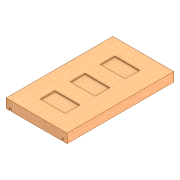
# Autodesk Inventor part: topplatform
Saved by Autodesk Inventor 2020 (Build 240168000, 168)
## iProperties
Created: 2021-06-22
Part Number: topplatform
Material: Generic
Document SubType Name: Modeling
Designer: Aidan Lee
Density: 1 g/cm^3
Appearance: Cherry - Natural Low Gloss
Author: Aidan Lee
Autodesk Inventor part; units mm, degrees
ref_plane "YZ Plane" through (0, 0, 0) normal (1, 0, 0) x (0, 1, 0)
ref_plane "XZ Plane" through (0, 0, 0) normal (0, 1, 0) x (-1, 0, 0)
ref_plane "XY Plane" through (0, 0, 0) normal (0, 0, 1) x (1, 0, 0)
sketch "Sketch1" plane through (0, 0, 0) normal (0, 0, 1) x (1, 0, 0)
  line L0 (0, 0) -> (120, 0)
  line L1 (120, 0) -> (120, 18)
  line L2 (120, 18) -> (0, 18)
  line L3 (0, 18) -> (0, 0)
  dimension "d0" = 18
  dimension "d1" = 120
  constraints: 8 end point, 2 parallel, 1 horizontal, 1 perpendicular
  measures "d0" distance of L2.end L0.start
  measures "d1" distance of L0.start L0.end
extrude "Extrusion1" add sketch "Sketch1" along normal blind 210
sketch "Sketch2" plane through (0, 0, 210) normal (0, 0, 1) x (1, 0, 0)
  line L0 (0, 0) -> (120, 0) projected
  line L1 (7, 0) -> (10, 0)
  line L2 (10, 0) -> (10, 5)
  line L3 (10, 5) -> (7, 5)
  line L4 (7, 5) -> (7, 0)
  line L5 (60, 0) -> (60, -17.5294) construction
  line L6 (113, 0) -> (110, 0)
  line L7 (110, 0) -> (110, 5)
  line L8 (110, 5) -> (113, 5)
  line L9 (113, 5) -> (113, 0)
  point P0 (110, 0)
  point P1 (113, 0)
  dimension "d4" = 3
  dimension "d5" = 5
  dimension "d26" = 100
  constraints: 18 end point, 4 symmetric about line, 2 parallel, 1 horizontal, 1 midpoint, 1 perpendicular, 1 point on line, 1 vertical
  measures "d4" distance of L2.end L3.end
  measures "d5" distance of L3.end L1.start
  measures "d26" distance between parallel lines of L7 L2
extrude "Extrusion2" cut sketch "Sketch2" against normal through all
sketch "Sketch3" plane through (0, 18, 0) normal (0, 1, 0) x (1, 0, 0)
  line L0 (35.5, -31.5) -> (84.5, -31.5)
  line L1 (84.5, -31.5) -> (84.5, -60.5)
  line L2 (84.5, -60.5) -> (35.5, -60.5)
  line L3 (35.5, -60.5) -> (35.5, -31.5)
  line L4 (35.5, -90.5) -> (84.5, -90.5)
  line L5 (84.5, -90.5) -> (84.5, -119.5)
  line L6 (84.5, -119.5) -> (35.5, -119.5)
  line L7 (35.5, -119.5) -> (35.5, -90.5)
  line L8 (35.5, -149.5) -> (84.5, -149.5)
  line L9 (84.5, -149.5) -> (84.5, -178.5)
  line L10 (84.5, -178.5) -> (35.5, -178.5)
  line L11 (35.5, -178.5) -> (35.5, -149.5)
  line L12 (0, 0) -> (0, -210) projected
  line L13 (120, 0) -> (0, 0) projected
  point P0 (0, -105)
  point P1 (35.5, -105)
  point P2 (60, 0)
  point P3 (60, -31.5)
  dimension "d9" = 29
  dimension "d10" = 49
  dimension "d13" = 59
  constraints: 24 end point, 4 midpoint, 2 parallel, 1 collinear, 1 horizontal, 1 horizontal alignment, 1 perpendicular, 1 vertical, 1 vertical alignment, 15 other
  measures "d9" distance of L0.end L1.end
  measures "d10" distance of L0.start L0.end
  measures "d13" distance of L0.start L4.start
extrude "Extrusion3" cut sketch "Sketch3" against normal blind 2
sketch "Sketch4" plane through (10, 0, 0) normal (0, -1, 0) x (1, 0, 0)
  line L0 (-10, 0) -> (-10, 210) projected
  line L1 (0, 0) -> (100, 0) projected
  line L2 (32.5, 106.5) -> (67.5, 106.5)
  line L3 (67.5, 106.5) -> (67.5, 103.5)
  line L4 (67.5, 103.5) -> (32.5, 103.5)
  line L5 (32.5, 103.5) -> (32.5, 106.5)
  point P0 (-10, 105)
  point P1 (32.5, 105)
  point P2 (50, 103.5)
  point P3 (50, 0)
  dimension "d20" = 3
  dimension "d21" = 35
  constraints: 8 end point, 4 midpoint, 2 parallel, 1 horizontal, 1 horizontal alignment, 1 perpendicular, 1 vertical alignment
  measures "d20" distance of L4.end L2.start
  measures "d21" distance of L2.start L2.end
extrude "Extrusion4" cut sketch "Sketch4" against normal blind 5
body "Solid1"
